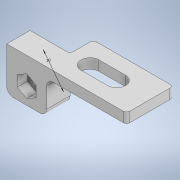
# Autodesk Inventor part: ystop
Saved by Autodesk Inventor 2022 (Build 260153000, 153)
## iProperties
Created: 2022-07-17
Part Number: ystop
Material: Genérico
Document SubType Name: Modeling
Designer: JK
Density: 1 g/cm^3
Appearance: Valor por defecto
Author: JK
Autodesk Inventor part; units mm, degrees
ref_plane "YZ Plane" through (0, 0, 0) normal (1, 0, 0) x (0, 1, 0)
ref_plane "XZ Plane" through (0, 0, 0) normal (0, 1, 0) x (-1, 0, 0)
ref_plane "XY Plane" through (0, 0, 0) normal (0, 0, 1) x (1, 0, 0)
sketch "Boceto1" plane through (0, 0, 0) normal (0, 1, 0) x (-1, 0, 0)
  line L0 (-12, 7) -> (12, 7)
  line L1 (12, 7) -> (12, -7)
  line L2 (12, -7) -> (-12, -7)
  line L3 (-12, -7) -> (-12, 7)
  line L4 (-12, 7) -> (12, -7) construction
  line L5 (12, 7) -> (-12, -7) construction
  circle A0 centre (6, 0) radius 2.7
  circle A1 centre (-2, 0) radius 2.7
  line L6 (6, 2.7) -> (-2, 2.7)
  line L7 (-2, 2.7) -> (-2, -2.7)
  line L8 (-2, -2.7) -> (6, -2.7)
  line L9 (6, -2.7) -> (6, 2.7)
  point P0 (0, 0)
  point P1 (0, 0)
  point P2 (6, -2.7)
  point P3 (-2, 2.7)
  dimension "d0" = 5.4
  dimension "d1" = 8
  dimension "d2" = 14
  dimension "d3" = 6
  dimension "d6" = 10
  constraints: 20 end point, 6 horizontal, 4 midpoint, 4 parallel, 2 perpendicular, 1 horizontal alignment, 6 other
  measures "d1" distance of L7.end L8.end
  measures "d2" distance between parallel lines of L2 L0
  measures "d3" distance from line of L1 point (6, 0)
  measures "d6" distance from line of L3 point (-2, 0)
extrude "Extrusión1" add sketch "Boceto1" along normal blind 3
sketch "Boceto2" plane through (0, 0, 0) normal (0, -1, 0) x (1, 0, 0)
  line L0 (-12, -7) -> (-12, 7) projected
  line L1 (-12, 7) -> (-24, 7)
  line L2 (-24, 7) -> (-24, 0)
  line L3 (-24, 0) -> (-12, 0)
  line L4 (-12, 0) -> (-12, 7)
  point P0 (0, 0)
  dimension "d7" = 12
  constraints: 8 end point, 2 parallel, 1 horizontal, 1 perpendicular
  measures "d7" distance between parallel lines of L0 L2
extrude "Extrusión2" add sketch "Boceto2" along normal blind 10 and the other way blind 3
fillet "Empalme1" radius 2 3 edges at (-12, 0, 3.5) (-12, -10, 3.5) (-24, -10, 3.5)
sketch "Boceto3" plane through (-12, 3, 0) normal (0, 0, -1) x (-1, 0, 0)
  circle A0 centre (6, -8) radius 1.65
  line L0 (10, -13) -> (2, -13) projected
  line L1 (12, -11) -> (12, 0) projected
  line L2 (-24, -3) -> (0, -3) projected
  point P0 (-12, -3)
  dimension "d13" = 3.3
  dimension "d15" = 6
  dimension "d24" = 5
  constraints: 1 centre point
  measures "d13" diameter of A0
  measures "d15" distance from line of A0.centre L1
  measures "d24" distance from line of L2 A0.centre
extrude "Extrusión3" cut sketch "Boceto3" against normal blind 8
sketch "Boceto4" plane through (-12, 3, 0) normal (0, 0, -1) x (-1, 0, 0)
  circle A0 centre (6, -8) radius 1.65 projected
  circle A1 centre (6, -8) radius 1.65 projected
  circle A2 centre (6, -8) radius 2.5
  point P0 (-12, -3)
  dimension "d18" = 5
  constraints: 1 centre point, 1 coincident
  measures "d18" diameter of A2
extrude "Extrusión4" add sketch "Boceto4" along normal blind 1
fillet "Empalme2" radius 1 1 edges at (-15.5, -5, 0)
fillet "Empalme3" radius 1 5 edges at (12, 1.5, 7) (12, 1.5, -7) (-12, 1.5, 0) (-12, 1.5, -7) (-11, 0, 0)
sketch "Boceto5" plane through (-18, -5, -1) normal (0, 0, -1) x (-1, 0, 0)
  circle A0 centre (0, 0) radius 1.65 projected
  circle A1 centre (0, 0) radius 5
  point P0 (-18, 5)
  dimension "d23" = 10
  constraints: 1 centre point, 1 coincident
  measures "d23" diameter of A1
sketch "Boceto6" plane through (-22, -10, 7) normal (0, 0, 1) x (1, 0, 0)
  circle A0 centre (4, 5) radius 2.8
  circle A1 centre (4, 5) radius 1.65 projected
  line L0 (4, 1.7668) -> (1.2, 3.3834)
  line L1 (1.2, 3.3834) -> (1.2, 6.6166)
  line L2 (1.2, 6.6166) -> (4, 8.2332)
  line L3 (4, 8.2332) -> (6.8, 6.6166)
  line L4 (6.8, 6.6166) -> (6.8, 3.3834)
  line L5 (6.8, 3.3834) -> (4, 1.7668)
  point P0 (22, 10)
  dimension "d25" = 5.6
  constraints: 12 end point, 1 centre point, 1 coincident, 1 concentric, 1 tangent, 1 vertical, 13 other
  measures "d25" diameter of A0
extrude "Extrusión5" cut sketch "Boceto6" against normal blind 3 contours A0 | L4 L5 A0 | A0 L3 L4 | A0 L2 L3 | L5 L0 A0 | A0 L1 L2 | L0 L1 A0 | A1
